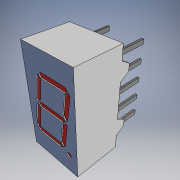
# Autodesk Inventor part: SA36-11EWA
Saved by Autodesk Inventor 2018 (Build 220112000, 112)
## iProperties
Created: 2020-04-20
Part Number: SA36-11EWA
Material: Všeobecné
Document SubType Name: Modeling
Designer: Jozko Mrkvicka
Density: 1 g/cm^3
Appearance: Výchozí
Author: Jozko Mrkvicka
Autodesk Inventor part; units mm, degrees
ref_plane "YZ Plane" through (0, 0, 0) normal (1, 0, 0) x (0, 1, 0)
ref_plane "XZ Plane" through (0, 0, 0) normal (0, 1, 0) x (-1, 0, 0)
ref_plane "XY Plane" through (0, 0, 0) normal (0, 0, 1) x (1, 0, 0)
sketch "Náčrt1" plane through (0, 0, 0) normal (0, 1, 0) x (-1, 0, 0)
  line L0 (0, 0) -> (13.97, 0)
  line L1 (13.97, 0) -> (13.97, -7.62)
  line L2 (13.97, -7.62) -> (0, -7.62)
  line L3 (0, -7.62) -> (0, 0)
  dimension "d0" = 13.97
  dimension "d1" = 7.62
  constraints: 8 end point, 2 parallel, 1 horizontal, 1 perpendicular
  measures "d0" distance of L1.end L2.end
  measures "d1" distance of L0.end L1.end
extrude "Vysunutí1" add sketch "Náčrt1" along normal blind 6.35
sketch "Náčrt3" plane through (0, 0, 0) normal (0, -1, 0) x (1, 0, 0)
  line L0 (-1.5875, -1.4287) -> (-2.2225, -1.4287)
  line L1 (-2.2225, -1.4287) -> (-2.2225, -1.1112)
  line L2 (-2.2225, -1.1112) -> (-1.5875, -1.1112)
  line L3 (-1.5875, -1.1112) -> (-1.5875, -1.4287)
  line L4 (-4.1275, -1.4287) -> (-4.7625, -1.4287)
  line L5 (-4.7625, -1.4287) -> (-4.7625, -1.1113)
  line L6 (-4.7625, -1.1113) -> (-4.1275, -1.1112)
  line L7 (-4.1275, -1.1112) -> (-4.1275, -1.4287)
  line L8 (-6.6675, -1.4287) -> (-7.3025, -1.4288)
  line L9 (-7.3025, -1.4288) -> (-7.3025, -1.1112)
  line L10 (-7.3025, -1.1112) -> (-6.6675, -1.1112)
  line L11 (-6.6675, -1.1112) -> (-6.6675, -1.4287)
  line L12 (-9.2075, -1.4287) -> (-9.8425, -1.4287)
  line L13 (-9.8425, -1.4287) -> (-9.8425, -1.1112)
  line L14 (-9.8425, -1.1112) -> (-9.2075, -1.1112)
  line L15 (-9.2075, -1.1112) -> (-9.2075, -1.4287)
  line L16 (-11.7475, -1.4287) -> (-12.3825, -1.4287)
  line L17 (-12.3825, -1.4287) -> (-12.3825, -1.1112)
  line L18 (-12.3825, -1.1112) -> (-11.7475, -1.1112)
  line L19 (-11.7475, -1.1112) -> (-11.7475, -1.4287)
  line L20 (-12.3825, -6.1913) -> (-11.7475, -6.1913)
  line L21 (-11.7475, -6.1913) -> (-11.7475, -6.5088)
  line L22 (-11.7475, -6.5088) -> (-12.3825, -6.5088)
  line L23 (-12.3825, -6.5088) -> (-12.3825, -6.1913)
  line L24 (-9.8425, -6.1913) -> (-9.2075, -6.1913)
  line L25 (-9.2075, -6.1913) -> (-9.2075, -6.5088)
  line L26 (-9.2075, -6.5088) -> (-9.8425, -6.5088)
  line L27 (-9.8425, -6.5088) -> (-9.8425, -6.1913)
  line L28 (-7.3025, -6.1913) -> (-6.6675, -6.1913)
  line L29 (-6.6675, -6.1913) -> (-6.6675, -6.5088)
  line L30 (-6.6675, -6.5088) -> (-7.3025, -6.5088)
  line L31 (-7.3025, -6.5088) -> (-7.3025, -6.1913)
  line L32 (-4.7625, -6.1913) -> (-4.1275, -6.1913)
  line L33 (-4.1275, -6.1913) -> (-4.1275, -6.5088)
  line L34 (-4.1275, -6.5088) -> (-4.7625, -6.5088)
  line L35 (-4.7625, -6.5088) -> (-4.7625, -6.1913)
  line L36 (-2.2225, -6.1913) -> (-1.5875, -6.1912)
  line L37 (-1.5875, -6.1912) -> (-1.5875, -6.5087)
  line L38 (-1.5875, -6.5087) -> (-2.2225, -6.5088)
  line L39 (-2.2225, -6.5088) -> (-2.2225, -6.1913)
  point P0 (0, 0)
  point P1 (-6.985, -1.27)
  point P2 (-6.985, -6.35)
  point P3 (-4.445, -1.27)
  point P4 (-9.525, -1.27)
  point P5 (-4.445, -6.35)
  point P6 (-9.525, -6.35)
  point P7 (-1.905, -1.27)
  point P8 (-4.445, -1.27)
  point P9 (-6.985, -1.27)
  point P10 (-9.525, -1.27)
  point P11 (-12.065, -1.27)
  point P12 (-12.065, -6.35)
  point P13 (-9.525, -6.35)
  point P14 (-6.985, -6.35)
  point P15 (-4.445, -6.35)
  point P16 (-1.905, -6.35)
  constraints: 80 end point, 20 parallel, 10 perpendicular
extrude "Vysunutí3" add sketch "Náčrt3" along normal blind 5.08
sketch "Náčrt4" plane through (0, 0, 0) normal (0, -1, 0) x (1, 0, 0)
  line L0 (-4.1275, -6.1913) -> (-4.1275, -6.5088) projected
  line L1 (-4.1275, -6.5088) -> (-4.7625, -6.5088) projected
  line L2 (-4.7625, -6.5088) -> (-4.7625, -6.1913) projected
  line L3 (-4.7625, -6.1913) -> (-4.1275, -6.1913) projected
  line L4 (-9.2075, -6.1913) -> (-9.2075, -6.5088) projected
  line L5 (-9.2075, -6.5088) -> (-9.8425, -6.5088) projected
  line L6 (-9.8425, -6.5088) -> (-9.8425, -6.1913) projected
  line L7 (-9.8425, -6.1913) -> (-9.2075, -6.1913) projected
  line L8 (-12.3825, -1.4287) -> (-12.3825, -1.1112) projected
  line L9 (-12.3825, -1.1112) -> (-11.7475, -1.1112) projected
  line L10 (-11.7475, -1.1112) -> (-11.7475, -1.4287) projected
  line L11 (-11.7475, -1.4287) -> (-12.3825, -1.4287) projected
  line L12 (-7.3025, -1.4288) -> (-7.3025, -1.1112) projected
  line L13 (-7.3025, -1.1112) -> (-6.6675, -1.1112) projected
  line L14 (-6.6675, -1.1112) -> (-6.6675, -1.4287) projected
  line L15 (-6.6675, -1.4287) -> (-7.3025, -1.4288) projected
  line L16 (-2.2225, -1.4287) -> (-2.2225, -1.1112) projected
  line L17 (-2.2225, -1.1112) -> (-1.5875, -1.1112) projected
  line L18 (-1.5875, -1.1112) -> (-1.5875, -1.4287) projected
  line L19 (-1.5875, -1.4287) -> (-2.2225, -1.4287) projected
  line L20 (-4.7625, -1.4287) -> (-4.7625, -1.1113) projected
  line L21 (-4.7625, -1.1113) -> (-4.1275, -1.1112) projected
  line L22 (-4.1275, -1.1112) -> (-4.1275, -1.4287) projected
  line L23 (-4.1275, -1.4287) -> (-4.7625, -1.4287) projected
  line L24 (-9.8425, -1.4287) -> (-9.8425, -1.1112) projected
  line L25 (-9.8425, -1.1112) -> (-9.2075, -1.1112) projected
  line L26 (-9.2075, -1.1112) -> (-9.2075, -1.4287) projected
  line L27 (-9.2075, -1.4287) -> (-9.8425, -1.4287) projected
  line L28 (-11.7475, -6.1913) -> (-11.7475, -6.5088) projected
  line L29 (-11.7475, -6.5088) -> (-12.3825, -6.5088) projected
  line L30 (-12.3825, -6.5088) -> (-12.3825, -6.1913) projected
  line L31 (-12.3825, -6.1913) -> (-11.7475, -6.1913) projected
  line L32 (-6.6675, -6.1913) -> (-6.6675, -6.5088) projected
  line L33 (-6.6675, -6.5088) -> (-7.3025, -6.5088) projected
  line L34 (-7.3025, -6.5088) -> (-7.3025, -6.1913) projected
  line L35 (-7.3025, -6.1913) -> (-6.6675, -6.1913) projected
  line L36 (-1.5875, -6.1912) -> (-1.5875, -6.5087) projected
  line L37 (-1.5875, -6.5087) -> (-2.2225, -6.5088) projected
  line L38 (-2.2225, -6.5088) -> (-2.2225, -6.1913) projected
  line L39 (-2.2225, -6.1913) -> (-1.5875, -6.1912) projected
  line L40 (0, 0) -> (-13.97, 0) projected
  line L41 (-1.5968, -0.3175) -> (-13.6525, -0.3175)
  line L42 (-0.3175, -1.5968) -> (-0.3175, -0.3175)
  line L43 (-0.3175, -7.3025) -> (-0.3175, -1.5968)
  line L44 (-13.6525, -0.3175) -> (-13.6525, -7.3025)
  line L45 (-0.3175, -7.3025) -> (-13.6525, -7.3025)
  line L46 (-1.5968, -0.3175) -> (-0.3175, -0.3175)
  constraints: 12 end point, 3 vertical, 2 horizontal, 1 parallel
extrude "Vysunutí4" cut sketch "Náčrt4" against normal blind 1.27
sketch "Náčrt5" plane through (0, 6.35, 0) normal (0, 1, 0) x (1, 0, 0)
  line L0 (-2.54, 4.8209) -> (-2.54, 1.2141)
  line L1 (-11.1963, 2.6568) -> (-11.1963, 6.2636)
  line L2 (-2.9007, 5.2417) -> (-2.54, 4.8209)
  line L3 (-2.9007, 5.2417) -> (-3.2614, 4.9411)
  line L4 (-2.54, 1.2141) -> (-2.9007, 0.9136)
  line L5 (-2.9007, 0.9136) -> (-3.2614, 1.3343)
  line L6 (-6.5075, 1.8754) -> (-6.8682, 1.5748)
  line L7 (-6.8682, 1.5748) -> (-7.2288, 1.9956)
  line L8 (-6.5075, 5.4822) -> (-6.8682, 5.903)
  line L9 (-6.8682, 5.903) -> (-7.2288, 5.6024)
  line L10 (-11.1963, 6.2636) -> (-10.8356, 6.5642)
  line L11 (-10.475, 6.1434) -> (-10.8356, 6.5642)
  line L12 (-3.4417, 4.9712) -> (-2.9894, 5.3481)
  line L13 (-3.4417, 1.3644) -> (-2.9908, 0.8384)
  line L14 (-10.475, 2.5366) -> (-10.8356, 2.236)
  line L15 (-10.8356, 2.236) -> (-11.1963, 2.6568)
  line L16 (-10.2946, 6.1134) -> (-10.7455, 6.6393)
  line L17 (-10.2904, 2.5059) -> (-10.738, 2.1222)
  line L18 (-10.7455, 6.6393) -> (-10.475, 6.8648)
  line L19 (-10.738, 2.1222) -> (-10.475, 1.8153)
  line L20 (-7.031, 1.4352) -> (-7.2288, 1.2742)
  line L21 (-6.7409, 1.4263) -> (-6.5075, 1.154)
  line L22 (-6.9864, 6.0449) -> (-7.2288, 6.3238)
  line L23 (-6.7033, 6.0404) -> (-6.5075, 6.2035)
  line L24 (-2.9908, 0.8384) -> (-3.2614, 0.613)
  line L25 (-2.9894, 5.3481) -> (-3.2497, 5.6606)
  line L26 (-3.2614, 1.3343) -> (-3.2614, 4.9411)
  line L27 (-3.4417, 1.3644) -> (-6.2642, 1.8348)
  line L28 (-7.2288, 1.9956) -> (-7.2288, 5.6024)
  line L29 (-6.2642, 1.8348) -> (-6.7409, 1.4263)
  line L30 (-10.475, 1.8153) -> (-7.2288, 1.2742)
  line L31 (-6.5075, 1.154) -> (-3.2614, 0.613)
  line L32 (-7.5895, 2.0557) -> (-7.031, 1.4352)
  line L33 (-3.4417, 4.9712) -> (-6.1468, 5.4221)
  line L34 (-6.5075, 5.4822) -> (-6.5075, 1.8754)
  line L35 (-3.2497, 5.6606) -> (-6.5075, 6.2035)
  line L36 (-6.7033, 6.0404) -> (-6.1468, 5.4221)
  line L37 (-7.4693, 5.6425) -> (-6.9864, 6.0449)
  line L38 (-7.4693, 5.6425) -> (-10.2946, 6.1134)
  line L39 (-7.2288, 6.3238) -> (-10.475, 6.8648)
  line L40 (-7.5895, 2.0557) -> (-10.2904, 2.5059)
  line L41 (-10.475, 2.5366) -> (-10.475, 6.1434)
  circle A0 centre (-11.43, 1.27) radius 0.3607
  constraints: 84 end point, 10 parallel, 6 point on line, 3 perpendicular, 1 centre point
extrude "Vysunutí5" cut sketch "Náčrt5" against normal blind 0.127
sketch "Náčrt6" plane through (0, 0, 0) normal (0, -1, 0) x (1, 0, 0)
  line L0 (-13.6525, -0.3175) -> (-0.3175, -0.3175) projected
  line L1 (-0.3175, -7.3025) -> (-13.6525, -7.3025) projected
  line L2 (0, 0) -> (-13.97, 0) projected
  line L3 (-1.905, 0) -> (-4.445, 0)
  line L4 (-4.445, 0) -> (-4.445, -0.3175)
  line L5 (-4.445, -0.3175) -> (-1.905, -0.3175)
  line L6 (-1.905, -0.3175) -> (-1.905, 0)
  line L7 (-9.525, 0) -> (-12.065, 0)
  line L8 (-12.065, 0) -> (-12.065, -0.3175)
  line L9 (-12.065, -0.3175) -> (-9.525, -0.3175)
  line L10 (-9.525, -0.3175) -> (-9.525, 0)
  line L11 (0, -7.62) -> (-13.97, -7.62) projected
  line L12 (-9.525, -7.3025) -> (-12.065, -7.3025)
  line L13 (-12.065, -7.3025) -> (-12.065, -7.62)
  line L14 (-12.065, -7.62) -> (-9.525, -7.62)
  line L15 (-9.525, -7.62) -> (-9.525, -7.3025)
  line L16 (0, -7.62) -> (-13.97, -7.62) projected
  line L17 (-1.905, -7.3025) -> (-4.445, -7.3025)
  line L18 (-4.445, -7.3025) -> (-4.445, -7.62)
  line L19 (-4.445, -7.62) -> (-1.905, -7.62)
  line L20 (-1.905, -7.62) -> (-1.905, -7.3025)
  point P0 (-9.525, -7.62)
  point P1 (-2.54, -7.62)
  point P2 (-8.255, -7.62)
  constraints: 32 end point, 9 point on line, 8 parallel, 4 horizontal, 4 perpendicular
extrude "Vysunutí6" add sketch "Náčrt6" along normal blind 1.27 contours L8 L2 L10 L0 | L4 L2 L6 L0 | L20 L11 L18 L1 | L15 L11 L13 L1
chamfer "Zkosení1" distance 0.762 distance2 1.27 1 edges at (-9.525, -1.27, -0.1587) measured on face at (-11.2183, -1.27, -0.1058)
chamfer "Zkosení2" distance 0.762 distance2 1.27 1 edges at (-4.445, -1.27, -0.1587) measured on face at (-3.5983, -1.27, -0.1058)
chamfer "Zkosení3" distance 0.762 distance2 1.27 1 edges at (-1.905, -1.27, -0.1587) measured on face at (-2.4978, -1.27, -0.2117)
chamfer "Zkosení4" distance 0.762 distance2 1.27 1 edges at (-12.065, -1.27, -0.1587) measured on face at (-11.4722, -1.27, -0.1058)
chamfer "Zkosení5" distance 0.762 distance2 1.27 1 edges at (-9.525, -1.27, -7.4613) measured on face at (-11.2183, -1.27, -7.4083)
chamfer "Zkosení6" distance 0.762 distance2 1.27 1 edges at (-12.065, -1.27, -7.4613) measured on face at (-11.4722, -1.27, -7.4083)
chamfer "Zkosení7" distance 0.762 distance2 1.27 1 edges at (-4.445, -1.27, -7.4613) measured on face at (-3.5983, -1.27, -7.4083)
chamfer "Zkosení8" distance 0.762 distance2 1.27 1 edges at (-1.905, -1.27, -7.4613) measured on face at (-2.4978, -1.27, -7.5142)
